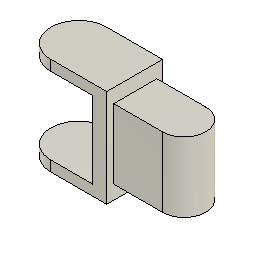
Trial3_v1 (Autodesk Fusion 360 design; units mm, degrees)
Autodesk Fusion 360 part; units mm, degrees
note: some values were not read from the file. Set by a fixed rule: which sketch regions a step uses.
sketch "Sketch1" plane through (0, 0, 0) normal (0, 0, 1) x (1, 0, 0)
  line L0 (0, 0) -> (0, 31.8988)
  line L1 (0, 31.8988) -> (70, 31.8988)
  line L2 (0, 0) -> (0, -30)
  line L3 (0, -30) -> (70, -30)
  arc A0 (70, -30) -> (70, 31.8988) centre (70, 0.9494) ccw
  dimension "d1" = 70
  dimension "d2" = 30
  dimension "d23" = 70
  constraint coincident L0.start L2.start
  constraint vertical L0
  constraint perpendicular L0 L1
  constraint parallel L0 L2
  constraint perpendicular L2 L3
  constraint tangent L3 A0
  measures "d1" distance of L0.end L1.end
  measures "d2" distance of L0.start L2.end
  measures "d23" distance of L2.end L3.end
extrude "Extrude1" add sketch "Sketch1" along normal mid plane 100
sketch "Sketch6" plane through (0, 0, 0) normal (0, 0, 1) x (1, 0, 0)
  line L0 (0, 0) -> (0, 40)
  line L1 (0, 0) -> (0, -40)
  line L2 (0, 40) -> (-80, 40)
  line L3 (-80, -40) -> (0, -40)
  line L4 (-80, -40) -> (-80, 40) construction
  arc A0 (-80, 40) -> (-80, -40) centre (-80, 0) ccw
  dimension "d24" = 40
  dimension "d25" = 40
  dimension "d42" = 80
  constraint coincident L0.start L1.start
  constraint vertical L0
  constraint parallel L0 L1
  constraint perpendicular L0 L2
  constraint perpendicular L1 L3
  constraint perpendicular L2 L4
  constraint midpoint L4 A0.centre
  measures "d24" distance of L0.start L0.end
  measures "d25" distance of L0.start L1.end
  measures "d42" distance of L1.end L3.start
extrude "Extrude5" add sketch "Sketch6" along normal mid plane 140
sketch "Sketch8" plane through (0, 0, 70) normal (0, 0, 1) x (-1, 0, 0)
  line L0 (0, 40) -> (0, -40)
  line L1 (0, -40) -> (80, -40)
  line L2 (80, 40) -> (0, 40)
  circle A0 centre (80, 0) radius 17.5 construction
  line L3 (80, 0) -> (80, -30) construction
  line L4 (80, 0) -> (48.1334, 0) construction
  line L5 (80, 0) -> (53.2858, -26.7142) construction
  circle A1 centre (67.6256, -12.3744) radius 2
  circle A2 centre (92.3744, -12.3744) radius 2
  circle A3 centre (92.3744, 12.3744) radius 2
  circle A4 centre (67.6256, 12.3744) radius 2
  arc A5 (80, -40) -> (80, 40) centre (80, 0) ccw
  dimension "d33" = 35
  dimension "d35" = 45
  dimension "d36" = 4
  dimension "d38" = 360
  constraint coincident A0.centre L3.start
  constraint vertical L3
  constraint perpendicular L3 L4
  constraint coincident A0 A1.centre
  constraint coincident L5 A1.centre
  measures "d33" diameter of A0
  measures "d35" angle of L4 L5
  measures "d36" diameter of A1
sketch "Sketch9" plane through (0, -40, 0) normal (0, -1, 0) x (1, 0, 0)
  line L0 (0, -70) -> (0, 70)
  line L1 (0, 70) -> (-80, 70)
  line L2 (-80, 70) -> (-80, -70)
  line L3 (-80, -70) -> (0, -70)
  line L4 (-160, 55) -> (-20, 55)
  line L5 (-20, 55) -> (-20, -55)
  line L6 (-20, -55) -> (-160, -55)
  line L7 (-160, -55) -> (-160, 55)
  dimension "d44" = 15
  dimension "d45" = 15
  dimension "d46" = 20
  constraint horizontal L4
  constraint vertical L5
  constraint horizontal L6
  constraint vertical L7
  measures "d44" distance of L1 L4
  measures "d45" distance of L3 L6
  measures "d46" distance of L0 L5
extrude "Extrude8" cut sketch "Sketch9" against normal blind 140 contours L2 L4 L6 L7 | L2 L4 L5 L6
sketch "Sketch10" plane through (0, 0, 0) normal (0, 1, 0) x (1, 0, 0)
  line L0 (70, -35) -> (70, -15) construction
  line L1 (70, 15) -> (70, 35) construction
  line L2 (70, 50) -> (70, -50)
  point P0 (70, -50)
  point P1 (70, 50)
  dimension "d49" = 20
  dimension "d50" = 20
  dimension "d51" = 30
  dimension "d52" = 15
  dimension "d53" = 15
  constraint vertical L0
  constraint collinear L0 L2
  measures "d49" distance of L0.start L0.end
  measures "d50" distance of L1.start L1.end
  measures "d51" distance of L0.end L1.start
  measures "d52" vertical distance of L0.start P0
  measures "d53" vertical distance of L1.end P1
scale "Scale1" factor 0.5 about (0, 40, 70) bodies 1
